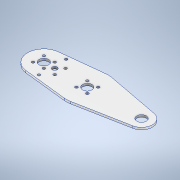
# Autodesk Inventor part: bean
Saved by Autodesk Inventor 2020 (Build 240168000, 168)
## iProperties
Created: 2019-12-28
Part Number: bean
Material: Aluminum 6061
Document SubType Name: Modeling
Designer: xj82b
Density: 2.7 g/cm^3
Appearance: Aluminum - Flat
Author: xj82b
Autodesk Inventor part; units mm, degrees
ref_plane "YZ Plane" through (0, 0, 0) normal (1, 0, 0) x (0, 1, 0)
ref_plane "XZ Plane" through (0, 0, 0) normal (0, 1, 0) x (-1, 0, 0)
ref_plane "XY Plane" through (0, 0, 0) normal (0, 0, 1) x (1, 0, 0)
sketch "Sketch1" plane through (0, 0, 0) normal (0, 1, 0) x (-1, 0, 0)
  line L0 (-28.6419, -11.7592) -> (-388.4279, -11.7592) construction
  arc A0 (-111.6419, 3.957) -> (-111.6419, -27.4755) centre (-108.6419, -11.7592) ccw
  arc A1 (37.9831, -35.6153) -> (37.9831, 12.0968) centre (35.3581, -11.7592) ccw
  line L1 (-25.2513, -42.5733) -> (37.9831, -35.6153)
  line L2 (-25.2513, 19.0548) -> (37.9831, 12.0968)
  line L3 (-34.4544, -42.2094) -> (-111.6419, -27.4755)
  line L4 (-111.6419, 3.957) -> (-34.4544, 18.691)
  arc A2 (-25.2513, 19.0548) -> (-34.4544, 18.691) centre (-28.6419, -11.7592) ccw
  arc A3 (-34.4544, -42.2094) -> (-25.2513, -42.5733) centre (-28.6419, -11.7592) ccw
  circle A4 centre (-108.6419, -11.7592) radius 7
  circle A5 centre (35.3581, -11.7592) radius 7
  circle A6 centre (-28.6419, -11.7592) radius 7
  circle A7 centre (27.3581, -3.7592) radius 2
  circle A8 centre (27.3581, -19.7592) radius 2
  circle A9 centre (43.3581, -19.7592) radius 2
  circle A10 centre (43.3581, -3.7592) radius 2
  circle A11 centre (35.3581, -11.7592) radius 11.3137 construction
  circle A12 centre (-108.6419, -11.7592) radius 43 construction
  circle A13 centre (-28.6419, -11.7592) radius 55 construction
  circle A14 centre (22.5928, -31.7592) radius 2
  circle A15 centre (22.5928, 8.2408) radius 2
  circle A16 centre (-36.6419, -19.7592) radius 2
  circle A17 centre (-20.6419, -19.7592) radius 2
  circle A18 centre (-20.6419, -3.7592) radius 2
  circle A19 centre (-36.6419, -3.7592) radius 2
  circle A20 centre (11.3581, -19.7592) radius 2
  circle A21 centre (11.3581, -3.7592) radius 2
  circle A22 centre (19.3581, -11.7592) radius 3.6
  dimension "d21" = 110
  dimension "d3" = 32
  dimension "d4" = 80
  dimension "d5" = 48
  dimension "d6" = 64
  dimension "d7" = 14
  dimension "d8" = 14
  dimension "d9" = 14
  dimension "d12" = 4
  dimension "d15" = 360
  dimension "d19" = 86
  dimension "d22" = 4
  dimension "d23" = 20
  dimension "d24" = 8
  dimension "d25" = 8
  dimension "d26" = 4
  dimension "d29" = 360
  dimension "d31" = 8
  dimension "d32" = 4
  dimension "d33" = 16
  dimension "d34" = 7.2
  dimension "d35" = 8
  constraints: 21 centre point, 10 end point, 8 point on circle, 8 tangent, 6 coincident, 4 horizontal alignment, 2 symmetric about line, 1 horizontal, 1 point on line, 27 other
  measures "d3" diameter of A0
  measures "d4" distance of L0.start A0.centre
  measures "d5" diameter of A1
  measures "d6" distance of A1.centre L0.start
  measures "d7" diameter of A4
  measures "d8" diameter of A5
  measures "d9" diameter of A6
  measures "d12" diameter of A7
  measures "d19" diameter of A12
  measures "d22" diameter of A14
  measures "d23" distance from line of L0 A14.centre
  measures "d24" distance from line of L0 A8.centre
  measures "d25" distance from line of L0 A9.centre
  measures "d26" diameter of A16
  measures "d31" distance from line of L0 A16.centre
  measures "d32" diameter of A20
  measures "d33" distance of A8.centre A20.centre
  measures "d34" diameter of A22
  measures "d35" horizontal distance of A22.centre A20.centre
extrude "Extrusion1" add sketch "Sketch1" along normal blind 3.175
body "Solid1"
